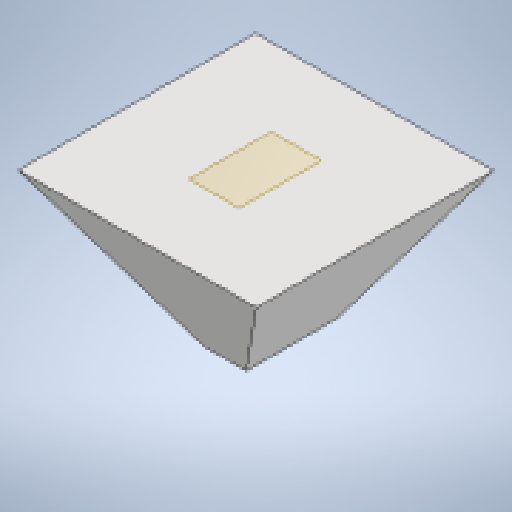
# Autodesk Inventor part: NDM-VOS dummy2
Saved by Autodesk Inventor 2025 (Build 290162010, 162A)
## iProperties
Created: 2024-07-24
Part Number: NDM-VOS dummy2
Material: Water
Document SubType Name: Modeling
Designer: admin
Mass: 1.15268e+06 g
Surface Area: 75607.2 cm^2
Volume: 1.15464e+06 cm^3
Density: 0.9983 g/cm^3
Appearance: Default
Author: admin
Autodesk Inventor part; units mm, degrees
ref_plane "YZ Plane" through (0, 0, 0) normal (1, 0, 0) x (0, 1, 0)
ref_plane "XZ Plane" through (0, 0, 0) normal (0, 1, 0) x (-1, 0, 0)
sketch "Sketch2" plane through (0, 0, 0) normal (0, 0, 1) x (1, 0, 0)
  line L0 (143.4494, -202.4371) -> (-143.4494, -202.4371)
  line L1 (-143.4494, -202.4371) -> (-143.4494, 411.0848)
  line L2 (-143.4494, 411.0848) -> (143.4494, 411.0848)
  line L3 (143.4494, 411.0848) -> (143.4494, -202.4371)
  line L4 (143.4494, -202.4371) -> (-143.4494, 411.0848) construction
  line L5 (-143.4494, -202.4371) -> (143.4494, 411.0848) construction
  point P0 (0, 0)
  point P1 (0, 104.3239)
  constraints: 12 end point, 2 midpoint, 2 parallel, 1 horizontal, 1 perpendicular, 1 vertical alignment
ref_plane "Work Plane1" through (0, 0, 1000) normal (0, 0, 1) x (1, 0, 0)
sketch "Sketch3" plane through (0, 0, 1000) normal (0, 0, 1) x (1, 0, 0)
  line L0 (807.3611, 799.8856) -> (-796.8238, 799.8856)
  line L1 (-796.8238, 799.8856) -> (-796.8238, -799.8856)
  line L2 (-796.8238, -799.8856) -> (807.3611, -799.8856)
  line L3 (807.3611, -799.8856) -> (807.3611, 799.8856)
  line L4 (807.3611, 799.8856) -> (-796.8238, -799.8856) construction
  line L5 (-796.8238, 799.8856) -> (807.3611, -799.8856) construction
  point P0 (0, 0)
  point P1 (5.2687, 0)
  constraints: 12 end point, 2 midpoint, 2 parallel, 1 horizontal, 1 perpendicular
loft "Loft1" add profiles "Sketch3", "Sketch2"
body "Solid2"
